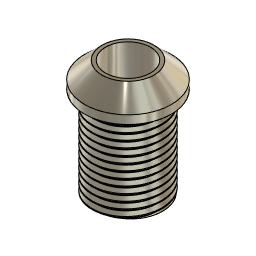
5mm led bezel (Autodesk Fusion 360 design; units mm, degrees)
Autodesk Fusion 360 part; units mm, degrees
sketch "Sketch1" plane through (0, 0, 0) normal (0, 0, 1) x (1, 0, 0)
  circle A0 centre (0, 0) radius 4
  circle A1 centre (0, 0) radius 3
  circle A2 centre (0, 0) radius 2.55
  dimension "d1" = 8
  dimension "d2" = 6
  dimension "d18" = 5.1
  constraint coincident A0.centre A1.centre
  constraint concentric A0 A1
  constraint concentric A0 A2
  measures "d1" diameter of A0
  measures "d2" diameter of A1
  measures "d18" diameter of A2
extrude "Extrude1" add sketch "Sketch1" along normal blind 9.7 contours A0 | A1
extrude "Extrude5" cut sketch "Sketch1" along normal blind 7.5 contours A1
chamfer "Chamfer3" distance 0.1 angle 45 1 edges at (-2.3774, 0.9221, 7.5)
sketch "Sketch2" plane through (0, 0, 9.7) normal (0, 0, 1) x (-1, 0, 0)
  circle A0 centre (0, 0) radius 4.125
  circle A1 centre (0, 0) radius 2.55
  dimension "d7" = 8.25
  constraint coincident A0.centre A1.centre
  measures "d7" diameter of A0
extrude "Extrude3" add sketch "Sketch2" along normal blind 0.5
ref_plane "WorkPlane1" through (0, 0, 13.1) normal (0, 0, 1) x (1, 0, 0)
sketch "Sketch3" plane through (0, 0, 13.1) normal (0, 0, 1) x (1, 0, 0)
  circle A0 centre (0, 0) radius 2.55
  circle A1 centre (0, 0) radius 2.95
  point P0 (3, 0)
  dimension "d22" = 0.4
sketch "Sketch4" plane through (0, 0, 10.2) normal (0, 0, 1) x (-1, 0, 0)
  circle A0 centre (0, 0) radius 4.925
  circle A1 centre (0, 0) radius 2.55
  dimension "d13" = 9.85
  constraint coincident A0.centre A1.centre
  measures "d13" diameter of A0
extrude "Extrude4" add sketch "Sketch4" along normal blind 1
sketch "Sketch7" plane through (0, 0, 11.2) normal (0, 0, 1) x (-1, 0, 0)
  circle A0 centre (0, 0) radius 2.55
  circle A1 centre (0, 0) radius 4.925
  line L0 (-2.55, 0) -> (-4.925, 0)
  circle A2 through (2.55, 0, 1.9) (-1.275, 2.2084, 1.9) (-1.275, -2.2084, 1.9)
  line L1 (-2.55, 0, 0) -> (-2.55, 0, 1.9)
  circle A3 through (2.95, 0, 1.9) (-1.475, 2.5548, 1.9) (-1.475, -2.5548, 1.9)
  line L2 (-2.55, 0, 1.9) -> (-2.95, 0, 1.9)
  line L3 (-2.95, 0, 1.9) -> (-4.925, 0, 0)
  line L4 (0, 0, 0) -> (0, 0, 1.9)
  point P0 (-2.55, 0)
  point P1 (-4.925, 0)
  constraint coincident P0 L0.start
  constraint coincident P1 L0.end
  constraint coincident A0.centre A1.centre
revolve "Revolve2" add sketch "Sketch7" angle 360 about axis through (0, 0, 11.2) along (0, 0, 1) contours L0 L1 L2 L3 in plane through (0, 0, 11.2) normal (0, -1, 0)
thread "Thread1" "ISO Metric profile 8.0 M8x0.75 6g" major diameter 7.908 minor diameter 7.0475 pitch 0.75 angle 60 modelled right hand crest width 0.1053 on face at (3.995, -0.1994, 6.4667) crest through (3.954, 0, -0.1875)
chamfer "Chamfer2" distance 0.05 angle 45 1 edges at (4.5917, 1.781, 10.2)
